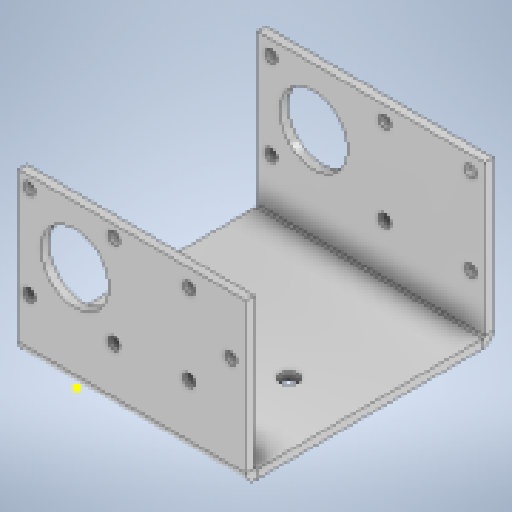
# Autodesk Inventor part: axis_25_bottom_frame
Saved by Autodesk Inventor 2025.2 (Build 292293000, 293)
## iProperties
Created: 2025-06-30
Part Number: axis_25_bottom_frame
Material: Aluminum 6061-AHC
Document SubType Name: Sheet Metal
Designer: LG
Density: 2.7 g/cm^3
Sheet Metal Rule: Default_mm
Appearance: Aluminum - Dark
Author: LG
Autodesk Inventor part; units mm, degrees
ref_plane "YZ Plane" through (0, 0, 0) normal (1, 0, 0) x (0, 1, 0)
ref_plane "XZ Plane" through (0, 0, 0) normal (0, 1, 0) x (-1, 0, 0)
ref_plane "XY Plane" through (0, 0, 0) normal (0, 0, 1) x (1, 0, 0)
sketch "Sketch1" plane through (0, 0, 0) normal (0, 1, 0) x (-1, 0, 0)
  line L0 (10.17, 20.25) -> (-29.83, 20.25)
  line L1 (-29.83, 20.25) -> (-29.83, -20.25)
  line L2 (-29.83, -20.25) -> (10.17, -20.25)
  line L3 (10.17, -20.25) -> (10.17, 20.25)
  point P0 (0, 0)
  dimension "d0" = 40.5
  dimension "d1" = 40
  dimension "d2" = 10.17
  dimension "d3" = 20.25
  measures "d0" distance of L2.end L0.start
  measures "d1" distance of L1.end L2.end
  measures "d2" distance from line of point (0, 0) L3
  measures "d3" distance from line of point (0, 0) L2
extrude "Plate1" add sketch "Sketch1" along normal blind 1.5
sketch "Sketch2" plane through (29.83, 0, 21.75) normal (0, 0, -1) x (-1, 0, 0)
  line L0 (40, 0) -> (0, 0)
  line L1 (0, 0) -> (0, 28.14)
  line L2 (0, 28.14) -> (40, 28.14)
  line L3 (40, 28.14) -> (40, 0)
  constraints: 8 end point
edge flange "Flange1" height 28.14 angle 90 thickness 1.5 bend radius 0.31 thickness toward (0, 0, -1) relief straight relief width 1.5 relief depth 0.75 corner gap 0.31 corner form 0 edges at (9.83, 1.5, 20.25) (9.83, 1.5, -20.25) wall of the first edge with corners at (-10.17, 0, 21.75) (29.83, 0, 21.75) (29.83, 28.14, 21.75) (-10.17, 28.14, 21.75)
bend "Bend1"
corner "Corner1"
sketch "Sketch6" plane through (-10.17, 28.14, 21.75) normal (0, 0, 1) x (1, 0, 0)
  point P0 (10.17, -28.14)
sketch "Sketch7" plane through (-10.17, 28.14, 21.75) normal (0, 0, 1) x (1, 0, 0)
  circle A0 centre (16.8, -2.07) radius 0.7835
  circle A1 centre (30.02, -3.07) radius 0.7835
  circle A2 centre (37.32, -10.07) radius 0.7835
  circle A3 centre (30.02, -17.07) radius 0.7835
  circle A4 centre (16.8, -18.07) radius 0.7835
  circle A5 centre (1.9, -2) radius 1
  circle A6 centre (1.9, -18.14) radius 1
  point P0 (10.17, -28.14)
  constraints: 7 centre point, 14 other
hole "Hole3" at (-8.27, 26.14, 21.75) at (-8.27, 10, 21.75) at (6.63, 26.07, 21.75) at (6.63, 10.07, 21.75) at (19.85, 25.07, 21.75) at (19.85, 11.07, 21.75) at (27.15, 18.07, 21.75) direction (0, 0, -1) diameter 2.1 depth 1.5
sketch "Sketch8" plane through (29.83, 28.14, -21.75) normal (0, 0, -1) x (-1, 0, 0)
  circle A0 centre (2.5, -2.545) radius 0.7835
  circle A1 centre (2.5, -17.595) radius 0.7835
  circle A2 centre (17.6, -2.545) radius 0.7835
  circle A3 centre (17.6, -17.595) radius 0.7835
  circle A4 centre (37.6, -2.545) radius 0.7835
  circle A5 centre (37.6, -17.595) radius 0.7835
  point P0 (29.83, -28.14)
  constraints: 6 centre point, 12 other
hole "Hole4" at (27.33, 25.595, -21.75) at (27.33, 10.545, -21.75) at (12.23, 25.595, -21.75) at (12.23, 10.545, -21.75) at (-7.77, 25.595, -21.75) at (-7.77, 10.545, -21.75) direction (0, 0, 1) diameter 2.1 depth 1.5
sketch "Sketch9" plane through (29.83, 28.14, -21.75) normal (0, 0, -1) x (-1, 0, 0)
  circle A0 centre (30.1, -10.07) radius 6
  point P0 (29.83, -28.14)
  constraints: 1 centre point, 2 other
extrude "Cut2" cut sketch "Sketch9" against normal blind 1.5
sketch "Sketch10" plane through (-10.17, 28.14, 21.75) normal (0, 0, 1) x (1, 0, 0)
  point P0 (10.17, -28.14)
sketch "Sketch11" plane through (-10.17, 28.14, 21.75) normal (0, 0, 1) x (1, 0, 0)
  point P0 (10.17, -28.14)
sketch "Sketch12" plane through (-10.17, 28.14, 21.75) normal (0, 0, 1) x (1, 0, 0)
  circle A0 centre (9.9, -10.07) radius 6
  point P0 (10.17, -28.14)
  constraints: 1 centre point, 2 other
extrude "Cut3" cut sketch "Sketch12" against normal blind 1.5
sketch "Sketch14" plane through (0, 0, 0) normal (0, -1, 0) x (1, 0, 0)
  circle A0 centre (0.78, 17.18) radius 1.55
  circle A1 centre (18.78, 17.18) radius 1.55
  circle A2 centre (18.78, 3.18) radius 1.55
  circle A3 centre (0.78, 3.18) radius 1.55
  point P0 (0, 0)
  constraints: 4 centre point, 8 other
extrude "Cut5" cut sketch "Sketch14" against normal blind 1.5
equation "\"d48\" = Thickness"
equation "\"d55\" = Thickness"
equation "\"d57\" = Thickness"
equation "\"d59\" = Thickness"
equation "\"d63\" = Thickness"
equation "\"d4\" = Thickness"
equation "\"d5\" = BendReliefWidth"
equation "\"d6\" = BendReliefDepth"
equation "\"d7\" = MinimumRemnant"
equation "\"d8\" = TransitionRadius"
equation "\"d11\" = BendRadius"
equation "\"d12\" = CornerReliefSize"
equation "\"d13\" = GapSize"
equation "\"d14\" = JacobiRadiusSize"
equation "\"BendReliefWidth\" = Thickness"
equation "\"BendReliefDepth\" = 0.5 * Thickness"
equation "\"CornerReliefSize\" = 4 * Thickness"
equation "\"MinimumRemnant\" = 2 * Thickness"
equation "\"TransitionRadius\" = BendRadius"
equation "\"JacobiRadiusSize\" = BendRadius"
equation "\"GapSize\" = Thickness"
equation "\"Thickness\" = 1.5"
equation "\"BendRadius\" = 0.31"
body "Solid1"
